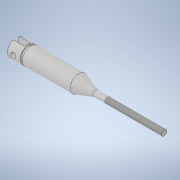
# Autodesk Inventor part: Anker
Saved by Autodesk Inventor 2021 (Build 250183000, 183)
## iProperties
Created: 2020-03-06
Part Number: Anker
Material: Generisch
Document SubType Name: Modeling
Designer: kaebi
Density: 1 g/cm^3
Appearance: Vorgabe
Author: kaebi
Autodesk Inventor part; units mm, degrees
ref_plane "YZ Plane" through (0, 0, 0) normal (1, 0, 0) x (0, 1, 0)
ref_plane "XZ Plane" through (0, 0, 0) normal (0, 1, 0) x (-1, 0, 0)
ref_plane "XY Plane" through (0, 0, 0) normal (0, 0, 1) x (1, 0, 0)
sketch "Skizze1" plane through (0, 0, 0) normal (0, 0, 1) x (1, 0, 0)
  line L0 (0, 0) -> (130, 0)
  line L1 (130, 0) -> (130, 2.5)
  line L2 (130, 2.5) -> (70, 2.5)
  line L3 (70, 2.5) -> (55, 7.5)
  line L4 (0, 7.5) -> (0, 0)
  line L5 (-57.0949, 0) -> (91.8524, 0)
  line L6 (-94.5139, 0) -> (167.419, 0) projected
  line L7 (0, -1.5) -> (0, 9) projected
  line L8 (11, 7.5) -> (11, 6.5)
  line L9 (11, 6.5) -> (13, 6.5)
  line L10 (13, 6.5) -> (13, 7.5)
  line L11 (55, 7.5) -> (13, 7.5)
  line L12 (11, 7.5) -> (0, 7.5)
  point P0 (0, 0)
  point P1 (0, -1.5)
  point P2 (0, 9)
  dimension "d0" = 130
  dimension "d1" = 5
  dimension "d3" = 55
  dimension "d4" = 15
  dimension "d5" = 11
  dimension "d6" = 2
  dimension "d7" = 1
  dimension "d8" = 15
  constraints: 22 end point, 6 perpendicular, 3 collinear, 2 horizontal, 2 parallel, 2 vertical, 1 other
  measures "d0" distance of L0.start L0.end
  measures "d1" diameter of L2 L5
  measures "d3" distance of L3.end L4.start
  measures "d4" horizontal distance of L2.end L3.end
  measures "d5" distance between parallel lines of L8 L4
  measures "d6" distance of L8.end L9.end
  measures "d7" distance of L9.end L10.end
  measures "d8" diameter of L12 L6
revolve "Umdrehung1" add sketch "Skizze1" angle 360 about axis through (-57.0949, 0, 0) along (1, 0, 0)
sketch "Skizze2" plane through (0, 0, 0) normal (0, 1, 0) x (-1, 0, 0)
  line L0 (0, 2.5) -> (-10, 2.5)
  line L1 (-10, 2.5) -> (-10, -2.5)
  line L2 (-10, -2.5) -> (0, -2.5)
  line L3 (0, -2.5) -> (0, 2.5)
  point P0 (0, 0)
  point P1 (0, 0)
  dimension "d10" = 10
  dimension "d11" = 5
  constraints: 8 end point, 2 parallel, 1 coincident, 1 horizontal, 1 midpoint, 1 perpendicular
  measures "d10" distance of L1.end L2.end
  measures "d11" distance of L0.end L1.end
extrude "Extrusion1" cut sketch "Skizze2" along normal through all both and the other way through all
sketch "Skizze3" plane through (0, 0, 0) normal (0, 0, 1) x (1, 0, 0)
  circle A0 centre (5, 0) radius 2.25
  line L0 (0, -7.0711) -> (0, 7.0711) projected
  point P0 (0, 0)
  point P1 (0, 0)
  dimension "d14" = 5
  dimension "d15" = 4.5
  constraints: 1 centre point, 1 horizontal alignment, 1 midpoint
  measures "d14" distance from line of L0 A0.centre
  measures "d15" diameter of A0
extrude "Extrusion2" cut sketch "Skizze3" along normal through all both and the other way through all
thread "Gewinde1" size "M5x0.8" class "6g" standard "ANSI Metric M Profile" length 50
